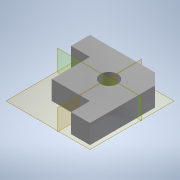
# Autodesk Inventor part: bevestiging deksel zonder moer
Saved by Autodesk Inventor 2021 (Build 250183000, 183)
## iProperties
Manager: Pierloot J.
Company: Emmaüs Bovenbouw Aalter
Created: 2021-01-26
Part Number: bevestiging deksel zonder moer
Material: S235
Catalog Web Link: http://emmausbovenbouw.op-weg.be/
Vendor: Emmaüsinstituut Bovenbouw Aalter
Document SubType Name: Modeling
Designer: iskhak.tchuytiyev
Engineer: Pierloot J.
Manufacturer: Standard
Standards Organization: Custom
Density: 7.86 g/cm^3
Appearance: Steel
Title: Algemene titel
Subject: Specifieke titel
Author: iskhak.tchuytiyev
Keywords: Ruwe Ø xxxxx
Comments: Opmerking
Autodesk Inventor part; units mm, degrees
sketch "Sketch1" plane through (0, 0, 0) normal (0, 0, 1) x (1, 0, 0)
  line L0 (-5.7775, 0) -> (5.7775, 0) construction
  line L1 (4.5, 7.5) -> (-12.5, 7.5)
  line L2 (-12.5, 7.5) -> (4.5, 7.5)
  line L3 (4.5, 7.5) -> (7.5, 4.5)
  line L4 (4.5, 7.5) -> (7.5, 4.5)
  line L5 (7.5, 4.5) -> (7.5, -12.5)
  line L6 (7.5, 4.5) -> (7.5, -12.5)
  line L7 (2.5, -12.5) -> (7.5, -12.5)
  line L8 (7.5, -12.5) -> (2.5, -12.5)
  line L9 (-7.5, -7.5) -> (2.5, -7.5)
  line L10 (2.5, -12.5) -> (2.5, -7.5)
  line L11 (2.5, -7.5) -> (-7.5, -7.5)
  line L12 (-7.5, 2.5) -> (-7.5, -7.5)
  line L13 (-7.5, -7.5) -> (-7.5, 2.5)
  line L14 (-7.5, 2.5) -> (-12.5, 2.5)
  line L15 (-7.5, 2.5) -> (-12.5, 2.5)
  line L16 (-12.5, 2.5) -> (-12.5, 7.5)
  constraints: 34 end point, 6 collinear, 3 perpendicular, 1 horizontal
extrude "Extrusion1" add sketch "Sketch1" along normal blind 5
sketch "Sketch2" plane through (0, 0, 5) normal (0, 0, 1) x (1, 0, 0)
  circle A0 centre (0, 0) radius 2.25
  dimension "d2" = 4.5
  constraints: 1 centre point, 1 coincident
  measures "d2" diameter of A0
extrude "Extrusion2" cut sketch "Sketch2" against normal blind 5
body "Solid1"
